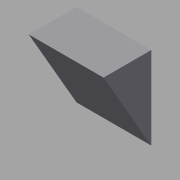
# Autodesk Inventor part: Wedge
Saved by Autodesk Inventor 2013 (Build 170138000, 138)
## iProperties
Created: 2013-01-25
Part Number: Wedge
Material: Generic
Document SubType Name: Modeling
Designer: Naphat
Density: 1 g/cm^3
Author: Naphat
Autodesk Inventor part; units mm, degrees
ref_plane "YZ Plane" through (0, 0, 0) normal (1, 0, 0) x (0, 1, 0)
ref_plane "XZ Plane" through (0, 0, 0) normal (0, 1, 0) x (-1, 0, 0)
ref_plane "XY Plane" through (0, 0, 0) normal (0, 0, 1) x (1, 0, 0)
sketch "Sketch1" plane through (0, 0, 0) normal (1, 0, 0) x (0, 1, 0)
  line L0 (0, 0) -> (505.932, 292.1)
  line L1 (0, 0) -> (584.2, 0) construction
  line L2 (505.932, 292.1) -> (505.932, 0)
  line L3 (505.932, 0) -> (0, 0)
  dimension "d0" = 584.2
  dimension "d1" = 30
  constraints: 8 end point, 1 equal length, 1 horizontal, 1 perpendicular, 1 vertical
  measures "d0" distance of L0.start L0.end
  measures "d1" angle of L1 L0
extrude "Extrusion1" add sketch "Sketch1" along normal blind 457.2
body "Solid1"
